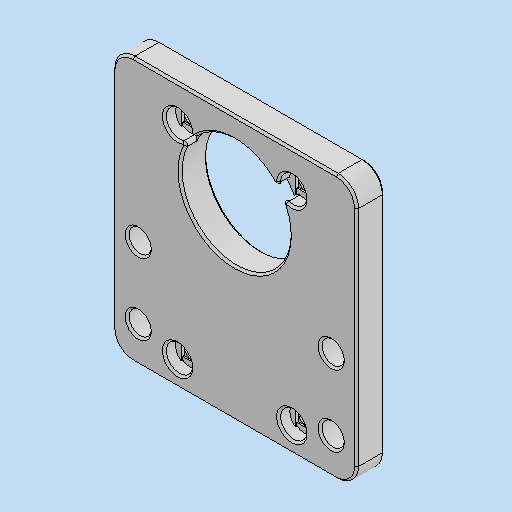
# Autodesk Inventor part: Motor-Plate
Saved by Autodesk Inventor 2025 (Build 290162000, 162)
## iProperties
Created: 2025-05-28
Part Number: Motor-Plate
Material: Generic
Document SubType Name: Modeling
Designer: kuzmin
Density: 1 g/cm^3
Appearance: Default
Mass: 9.35418 g
Surface Area: 53.1158 cm^2
Volume: 9.35418 cm^3
Author: kuzmin
Autodesk Inventor part; units mm, degrees
ref_plane "YZ Plane" through (0, 0, 0) normal (1, 0, 0) x (0, 1, 0)
ref_plane "XZ Plane" through (0, 0, 0) normal (0, 1, 0) x (-1, 0, 0)
ref_plane "XY Plane" through (0, 0, 0) normal (0, 0, 1) x (1, 0, 0)
sketch "Sketch1" plane through (0, 0, 0) normal (0, 0, 1) x (1, 0, 0)
  line L0 (-24, 26) -> (24, 26)
  line L1 (24, 26) -> (24, -26)
  line L2 (24, -26) -> (-24, -26)
  line L3 (-24, -26) -> (-24, 26)
  point P0 (0, 0)
  point P1 (0, 26)
  point P2 (24, 0)
  dimension "d0" = 48
  dimension "d1" = 52
  constraints: 8 end point, 2 midpoint, 2 parallel, 1 horizontal, 1 horizontal alignment, 1 perpendicular, 1 vertical alignment
  measures "d0" distance of L1.end L2.end
  measures "d1" distance of L0.end L1.end
extrude "Extrusion1" add sketch "Sketch1" along normal blind 5.5
sketch "Sketch4" plane through (0, 0, 5.5) normal (0, 0, 1) x (1, 0, 0)
  line L0 (-11.25, 18.85) -> (11.25, 18.85) construction
  line L1 (11.25, 18.85) -> (11.25, -21.15) construction
  line L2 (11.25, -21.15) -> (-11.25, -21.15) construction
  line L3 (-11.25, -21.15) -> (-11.25, 18.85) construction
  line L4 (24, 26) -> (-24, 26) construction
  point P0 (0, 0)
  point P1 (0, 18.85)
  dimension "d9" = 7.15
  dimension "d10" = 22.5
  dimension "d11" = 40
  constraints: 8 end point, 4 coincident, 2 parallel, 1 horizontal, 1 midpoint, 1 perpendicular, 1 vertical alignment
  measures "d9" distance between parallel lines of L4 L0
  measures "d10" distance of L0.start L0.end
  measures "d11" distance of L0.end L1.end
hole "Hole1" at (-11.25, 18.85, 5.5) at (11.25, 18.85, 5.5) at (-11.25, -21.15, 5.5) at (11.25, -21.15, 5.5) direction (0, 0, -1) diameter 3 end through all counterbore diameter 5.2 counterbore depth 2.8
sketch "Sketch5" plane through (0, 0, 5.5) normal (0, 0, 1) x (1, 0, 0)
  circle A0 centre (0, 11.1) radius 10.75
  line L0 (24, 26) -> (-24, 26) projected
  circle A1 centre (11.25, 18.85) radius 2.6 projected
  point P0 (0, 0)
  dimension "d19" = 21.5
  dimension "d24" = 7.75
  constraints: 1 centre point, 1 vertical alignment
  measures "d19" diameter of A0
  measures "d24" vertical distance of A0.centre A1.centre
extrude "Extrusion4" cut sketch "Sketch5" against normal through all contours A0
fillet "Fillet1" radius 4 4 edges at (24, -26, 2.75) (-24, -26, 2.75) (-24, 26, 2.75) (24, 26, 2.75)
sketch "Sketch6" plane through (0, 0, 5.5) normal (0, 0, 1) x (1, 0, 0)
  line L0 (-19, -5) -> (19, -5) construction
  line L1 (19, -5) -> (19, -19) construction
  line L2 (19, -19) -> (-19, -19) construction
  line L3 (-19, -19) -> (-19, -5) construction
  line L4 (-20, -26) -> (20, -26) projected
  point P0 (0, 0)
  point P1 (0, -4)
  point P2 (0, -5)
  dimension "d36" = 38
  dimension "d37" = 14
  dimension "d70" = 7
  constraints: 8 end point, 3 coincident, 2 parallel, 2 vertical alignment, 1 horizontal, 1 midpoint, 1 perpendicular
  measures "d36" distance of L0.start L0.end
  measures "d37" distance of L2.end L0.start
  measures "d70" distance between parallel lines of L4 L2
hole "Hole2" at (-19, -5, 5.5) at (19, -5, 5.5) at (-19, -19, 5.5) at (19, -19, 5.5) direction (0, 0, -1) diameter 4.4 end through all
sketch "Sketch7" plane through (0, 0, 0) normal (0, 0, -1) x (-1, 0, 0)
  line L0 (-11.5, 15.8) -> (-14.5, 15.8) projected
  arc A0 (-11.5, 15.8) -> (-8.2, 19.1) centre (-11.5, 19.1) ccw projected
  line L1 (-8.2, 22.1) -> (-8.2, 19.1) projected
  line L2 (-12.3, 22.1) -> (-8.2, 22.1) projected
  line L3 (-14.5, 19.9) -> (-12.3, 22.1) projected
  line L4 (-14.5, 15.8) -> (-14.5, 19.9) projected
  circle A1 centre (-11.25, 18.85) radius 1.45 projected
  line L5 (8.2, 19.1) -> (8.2, 22.1) projected
  arc A2 (8.2, 19.1) -> (11.5, 15.8) centre (11.5, 19.1) ccw projected
  line L6 (14.5, 15.8) -> (11.5, 15.8) projected
  line L7 (14.5, 19.9) -> (14.5, 15.8) projected
  line L8 (12.3, 22.1) -> (14.5, 19.9) projected
  line L9 (8.2, 22.1) -> (12.3, 22.1) projected
  circle A3 centre (11.25, 18.85) radius 1.45 projected
  line L10 (11.5, -18.1) -> (14.5, -18.1) projected
  arc A4 (11.5, -18.1) -> (8.2, -21.4) centre (11.5, -21.4) ccw projected
  line L11 (8.2, -24.4) -> (8.2, -21.4) projected
  line L12 (12.3, -24.4) -> (8.2, -24.4) projected
  line L13 (14.5, -22.2) -> (12.3, -24.4) projected
  line L14 (14.5, -18.1) -> (14.5, -22.2) projected
  circle A5 centre (11.25, -21.15) radius 1.45 projected
  line L15 (-8.2, -21.4) -> (-8.2, -24.4) projected
  arc A6 (-8.2, -21.4) -> (-11.5, -18.1) centre (-11.5, -21.4) ccw projected
  line L16 (-14.5, -18.1) -> (-11.5, -18.1) projected
  line L17 (-14.5, -22.2) -> (-14.5, -18.1) projected
  line L18 (-12.3, -24.4) -> (-14.5, -22.2) projected
  line L19 (-8.2, -24.4) -> (-12.3, -24.4) projected
  circle A7 centre (-11.25, -21.15) radius 1.45 projected
  point P0 (0, 0)
extrude "Extrusion5" add sketch "Sketch7" along normal blind 2.9
sketch "Sketch8" plane through (-11.25, 18.85, 2.7) normal (0, 0, 1) x (1, 0, 0)
  circle A0 centre (0, 0) radius 2.6 projected
  circle A1 centre (0, 0) radius 1.5 projected
  line L0 (-2.1237, 1.5) -> (2.1237, 1.5)
  line L1 (-2.1237, -1.5) -> (2.1237, -1.5)
  line L2 (1.5, 2.1237) -> (1.5, -2.1237)
  line L3 (-1.5, 2.1237) -> (-1.5, -2.1237)
  circle A2 centre (0, 0) radius 1.5 projected
  point P0 (11.25, -18.85)
  constraints: 8 end point, 4 tangent, 1 horizontal, 1 parallel, 1 perpendicular, 1 vertical, 9 other
extrude "Extrusion6" add sketch "Sketch8" along normal blind 0.3 contours L0 L2 A0 | A0 L2 L1 | L2 L0 L3 A0 | A0 L3 L1 L2 | L3 L0 A0 | A0 L1 L3
extrude "Extrusion7" add sketch "Sketch8" along normal blind 0.6 contours A0 L1 L2 L0 | L0 L2 A0 | A0 L2 L1 | L3 L0 A0 | A0 L1 L3 | L0 L3 L1 A0
pattern_linear "Rectangular Pattern1" count 2 spacing 40 along (0, -1, 0) count 2 spacing 22.5 along (1, 0, 0) of "Extrusion7", "Extrusion6"
sketch "Sketch9" plane through (0, 0, 5.5) normal (0, 0, 1) x (1, 0, 0)
  circle A0 centre (-11.25, 18.85) radius 2.6 projected
  line L0 (-8.9051, 17.727) -> (-8.6164, 17.5281)
  arc A1 (-9.75, 16.7263) -> (-9.75, 20.9737) centre (-11.25, 18.85) ccw projected
  arc A2 (-9.0764, 16.8603) -> (9.0764, 16.8603) centre (0, 11.1) ccw projected
  line L1 (-9.3651, 17.0591) -> (-9.0764, 16.8603)
  line L2 (-11.25, 18.85) -> (0, 11.1) construction
  circle A3 centre (0, 11.1) radius 10.75 projected
  line L3 (-8.6164, 17.5281) -> (-9.0764, 16.8603) construction
  point P0 (0, 0)
  point P1 (-8.8464, 17.1942)
  constraints: 8 end point, 3 point on circle, 2 parallel, 1 coincident, 1 midpoint, 1 point on line
extrude "Extrusion8" cut sketch "Sketch9" against normal up to surface (2.2 mm away) contours L0 A3 L1 A0
mirror "Mirror1" about plane through (0, 0, 0) normal (1, 0, 0) of "Extrusion8"
fillet "Fillet3" radius 0.5 8 edges at (-8.6164, 17.5281, 4.4) (-8.9051, 17.727, 4.4) (-9.0764, 16.8603, 4.4) (-9.3651, 17.0591, 4.4) (8.6164, 17.5281, 4.4) (8.9051, 17.727, 4.4) (9.0764, 16.8603, 4.4) (9.3651, 17.0591, 4.4)
chamfer "Chamfer1" distance 0.4 angle 45 31 edges at (0, 26, 5.5) (-22.8284, 24.8284, 5.5) (-24, 0, 5.5) (-22.8284, -24.8284, 5.5) (0, -26, 5.5) (22.8284, -24.8284, 5.5) (24, 0, 5.5) (22.8284, 24.8284, 5.5) (0, 26, 0) (-22.8284, 24.8284, 0) (-24, 0, 0) (-22.8284, -24.8284, 0) (0, -26, 0) (22.8284, -24.8284, 0) (24, 0, 0) (22.8284, 24.8284, 0) (-19, -2.8, 0) (-19, -16.8, 0) (19, -16.8, 0) (19, -2.8, 0) (0, 21.85, 5.5) (-2.3769, 0.6161, 5.5) (10.4839, 13.4769, 5.5) (13.3911, 20.325, 5.5) (11.25, -18.55, 5.5) (-11.25, -18.55, 5.5) (-13.3911, 20.325, 5.5) (-19, -2.8, 5.5) (19, -2.8, 5.5) (19, -16.8, 5.5) (-19, -16.8, 5.5)
fillet "Fillet2" radius 1 16 edges at (14.5, 15.8, -1.45) (8.2, 22.1, -1.45) (12.3, 22.1, -1.45) (14.5, 19.9, -1.45) (-14.5, 15.8, -1.45) (-14.5, 19.9, -1.45) (-12.3, 22.1, -1.45) (-8.2, 22.1, -1.45) (-14.5, -22.2, -1.45) (-12.3, -24.4, -1.45) (-8.2, -24.4, -1.45) (-14.5, -18.1, -1.45) (8.2, -24.4, -1.45) (12.3, -24.4, -1.45) (14.5, -22.2, -1.45) (14.5, -18.1, -1.45)
chamfer "Chamfer3" distance 0.5 angle 45 3 edges at (0, 21.85, 0) (10.3231, 14.0992, 0) (-2.9992, 0.7769, 0)
chamfer "Chamfer4" distance 0.4 angle 45 40 edges at (13.4, 21, -2.9) (14.4239, 19.8685, -2.9) (14.5, 18.1429, -2.9) (14.2071, 16.0929, -2.9) (12.5, 15.8, -2.9) (9.1665, 16.7665, -2.9) (8.2, 20.1, -2.9) (8.4929, 21.8071, -2.9) (10.5429, 22.1, -2.9) (12.2685, 22.0239, -2.9) (-9.1665, 16.7665, -2.9) (-12.5, 15.8, -2.9) (-14.2071, 16.0929, -2.9) (-14.5, 18.1429, -2.9) (-14.4239, 19.8685, -2.9) (-13.4, 21, -2.9) (-12.2685, 22.0239, -2.9) (-10.5429, 22.1, -2.9) (-8.4929, 21.8071, -2.9) (-8.2, 20.1, -2.9) (-9.1665, -19.0665, -2.9) (-8.2, -22.4, -2.9) (-8.4929, -24.1071, -2.9) (-10.5429, -24.4, -2.9) (-12.2685, -24.3239, -2.9) (-13.4, -23.3, -2.9) (-14.4239, -22.1685, -2.9) (-14.5, -20.4429, -2.9) (-14.2071, -18.3929, -2.9) (-12.5, -18.1, -2.9) (9.1665, -19.0665, -2.9) (12.5, -18.1, -2.9) (14.2071, -18.3929, -2.9) (14.5, -20.4429, -2.9) (14.4239, -22.1685, -2.9) (13.4, -23.3, -2.9) (12.2685, -24.3239, -2.9) (10.5429, -24.4, -2.9) (8.4929, -24.1071, -2.9) (8.2, -22.4, -2.9)
chamfer "Chamfer5" distance 0.3 angle 45 20 edges at (14.4239, -22.1685, 0) (13.4, -23.3, 0) (12.2685, -24.3239, 0) (10.5429, -24.4, 0) (8.4929, -24.1071, 0) (8.2, -22.4, 0) (9.1665, -19.0665, 0) (12.5, -18.1, 0) (14.2071, -18.3929, 0) (14.5, -20.4429, 0) (-8.4929, -24.1071, 0) (-10.5429, -24.4, 0) (-12.2685, -24.3239, 0) (-13.4, -23.3, 0) (-14.4239, -22.1685, 0) (-14.5, -20.4429, 0) (-14.2071, -18.3929, 0) (-12.5, -18.1, 0) (-9.1665, -19.0665, 0) (-8.2, -22.4, 0)
equation "\"d19\" = hole"
equation "\"hole\" = 21.5"
equation "\"width\" = 48"
equation "\"hight\" = 52"
body "Solid1"
